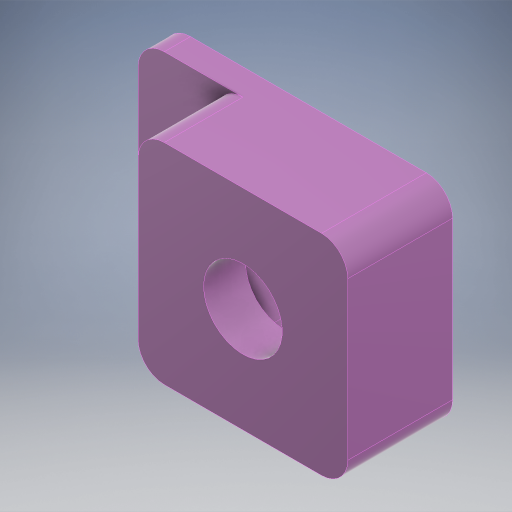
# Autodesk Inventor part: Передние основные крепежи
Saved by Autodesk Inventor 2023 (Build 270158000, 158)
## iProperties
Created: 2023-03-26
Part Number: Передние основные крепежи
Material: Типовые
Document SubType Name: Modeling
Designer: Admin
Density: 1 g/cm^3
Appearance: По умолчанию
Author: Admin
Autodesk Inventor part; units mm, degrees
ref_plane "YZ Plane" through (0, 0, 0) normal (1, 0, 0) x (0, 1, 0)
ref_plane "XZ Plane" through (0, 0, 0) normal (0, 1, 0) x (-1, 0, 0)
ref_plane "XY Plane" through (0, 0, 0) normal (0, 0, 1) x (1, 0, 0)
sketch "Эскиз1" plane through (0, 0, 0) normal (0, 0, 1) x (1, 0, 0)
  line L0 (6, -8) -> (-6, -8)
  line L1 (-8, -8) -> (-8, 6)
  line L2 (-6, 8) -> (6, 8)
  line L3 (8, 6) -> (8, -6)
  line L4 (-8, 8) -> (-12, 8)
  line L5 (-14, 6) -> (-14, -6)
  line L6 (-12, -8) -> (-8, -8)
  line L7 (-8, -6) -> (-8, 8)
  circle A0 centre (0, 0) radius 3
  line L8 (-2.8579, -4.95) -> (-5.7158, 0)
  line L9 (-5.7158, 0) -> (-2.8579, 4.95)
  line L10 (-2.8579, 4.95) -> (2.8579, 4.95)
  line L11 (2.8579, 4.95) -> (5.7158, 0)
  line L12 (5.7158, 0) -> (2.8579, -4.95)
  line L13 (2.8579, -4.95) -> (-2.8579, -4.95)
  arc A1 (-14, -6) -> (-12, -8) centre (-12, -6) ccw
  arc A2 (-12, 8) -> (-14, 6) centre (-12, 6) ccw
  arc A3 (-6, 8) -> (-8, 6) centre (-6, 6) ccw
  arc A4 (-8, -6) -> (-6, -8) centre (-6, -6) ccw
  arc A5 (6, -8) -> (8, -6) centre (6, -6) ccw
  arc A6 (8, 6) -> (6, 8) centre (6, 6) ccw
  line L14 (-6, -8) -> (-8, -8)
  line L15 (-6, 8) -> (-8, 8)
  point P0 (8, 0)
  point P1 (0, -8)
  point P2 (-8, -6)
  dimension "d0" = 6
  dimension "Fit1" = 16
  dimension "Fit2" = 22
  dimension "d3" = 2
  dimension "d4" = 16
  dimension "Nut_fit" = 9.9
  constraints: 33 end point, 13 tangent, 12 point on circle, 7 centre point, 5 equal radius, 4 horizontal, 4 parallel, 4 point on line, 2 coincident, 2 midpoint, 2 perpendicular, 1 horizontal alignment, 1 vertical alignment, 13 other
  measures "d0" diameter of A0
  measures "Fit1" distance between parallel lines of L3 L1
  measures "Fit2" distance between parallel lines of L3 L5
  measures "d3" radius of A1
  measures "d4" distance between parallel lines of L2 L0
  measures "Nut_fit" distance between parallel lines of L13 L10
extrude "Выдавливание1" add sketch "Эскиз1" along normal blind 6 contours L0 A4 L1 A3 L2 A6 L3 A5 | A0 | L8 L9 L10 L11 L12 L13
extrude "Выдавливание2" add sketch "Эскиз1" against normal blind 2 contours L0 A4 L1 A3 L2 A6 L3 A5 | L14 L1 A4 | L1 L6 A1 L5 A2 L4 L7 | L7 L15 A3
extrude "Выдавливание3" cut sketch "Эскиз1" along normal blind 2.8 contours A0 | L8 L9 L10 L11 L12 L13
extrude "Выдавливание4" cut sketch "Эскиз1" along normal through all contours A0
